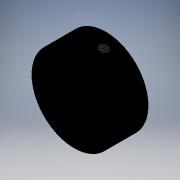
# Autodesk Inventor part: SCHUNK-Flansch IP 40 ERD
Saved by Autodesk Inventor 2017.3 (Build 213256000, 256)
## iProperties
Part Number: SCHUNK-Flansch IP 40 ERD
Material: Generic
Catalog Web Link: www.cadenas.de
Description: Flansch ERD-Miniature rotary unit
Vendor: SCHUNK
Document SubType Name: Modeling
Designer: partserver
Manufacturer: SCHUNK
Mass: 46.2323 g
Surface Area: 96.2708 cm^2
Volume: 46.2323 cm^3
Density: 1 g/cm^3
Appearance: PSOLRGB-0-0-0
Category: PARTsolutions
Company: SCHUNK
Title: SCHUNK-Flansch IP 40 ERD
Author: Cadenas PARTsolutions
Comments: Miniature rotary unit
PSOL_IDENT_0: {$CADENAS_DATA\23d-libs\schunk\greifsysteme\drehmodule\drehmodule_elektrisch\schwenkeinheiten\miniat
PSOL_IDENT_1: ur_schwenkeinheiten\erd_welle.prj},193 {VTYP=3D},{NB=SCHUNK-Flansch IP 40 ERD},{LINA=SCHUNK-Flansch
PSOL_IDENT_2: IP 40 ERD},{NN=Flansch ERD},{DATE=23.04.2020 15:23:31},{GEOMDATE=04.12.2019 08:06:04},{VERSION=},{LI
PSOL_IDENT_3: NEID=20},{WBVAR=},{WBNUMERIC=}  {NB=SCHUNK-Flansch IP 40 ERD},{LINA=SCHUNK-Flansch IP 40 ERD},{KT=DU
PSOL_IDENT_4: MMY},{TYP=Flansch IP 40},{KD1=55.000},{KD2=25.000},{KH1=20.500},{KH2=2.000},{BA1=28.300},{BA2=20.000
PSOL_IDENT_5: },{BA3=11.000},{BD1=5.000},{BD2=5.000},{BD3=10.000},{BD4=4.200},{BD5=2.500},{BT1=11.000},{BT2=5.000}
PSOL_IDENT_6: ,{BT3=0.700},{BT4=2.500},{BA4=20.500},{BA5=12.500},{BD6=10.000},{BD7=7.000},{BT6=0.500},{BT7=5.000},
PSOL_IDENT_7: {BW=15.000},{SBD=2.500},{SBW=4.000},{SBA1=8.500},{SBA2=22.700},{SBA3=13.000},{SBT1=10.400},{SBT2=22.
PSOL_IDENT_8: 900},{TYP1=40.000}
NB: SCHUNK-Flansch IP 40 ERD
NN: Flansch ERD
NT: Miniature rotary unit
NBSYN: SCHUNK-$TYP. ERD
LINA: SCHUNK-Flansch IP 40 ERD
CATALOG: SCHUNK
TYP: Flansch IP 40
KD1: 55
KD2: 25
KH1: 20.5
KH2: 2
BA1: 28.3
BA2: 20
BA3: 11
BD1: 5
BD2: 5
BD3: 10
BD4: 4.2
BD5: 2.5
BT1: 11
BT2: 5
BT3: 0.7
BT4: 2.5
BA4: 20.5
BA5: 12.5
BD6: 10
BD7: 7
BT6: 0.5
BT7: 5
BW: 15
SBD: 2.5
SBW: 4
SBA1: 8.5
SBA2: 22.7
SBA3: 13
SBT1: 10.4
SBT2: 22.9
TYP1: 40
SUPPLIER: SCHUNK
ARTICLENO: SCHUNK-Flansch IP 40 ERD
BOMINFO: SCHUNK-Flansch IP 40 ERD
CREATOR: CADENAS GmbH
Autodesk Inventor part; units mm, degrees
sketch "Sketch_1" plane through (0, 0, 0) normal (0, 0, 1) x (1, 0, 0)
  line L0 (0, 0) -> (0, 20)
  line L1 (0, 18.5) -> (12.5, 18.5)
  line L2 (12.5, 18.5) -> (12.5, 20.2)
  line L3 (12.5, 20.2) -> (12.8, 20.5)
  line L4 (12.8, 20.5) -> (27.5, 20.5)
  line L5 (27.5, 20.5) -> (27.5, 0)
  line L6 (27.5, 0) -> (0, 0)
  line L7 (0, 0) -> (0, 18.5)
  constraints: 16 end point
revolve "Revolution1" add sketch "Sketch_1" angle 360 about axis through (0, 0, 0) along (0, -1, 0)
sketch "Sketch_2" plane through (0, 0, 0) normal (1, 0, 0) x (0, 1, 0)
  line L0 (18.5, 5.5) -> (14.5489, 5.5)
  line L1 (14.5489, 5.5) -> (15.3, 6.75)
  line L2 (15.3, 6.75) -> (17.6, 6.75)
  line L3 (17.6, 6.75) -> (17.8, 6.95)
  line L4 (17.8, 6.95) -> (17.8, 7.4)
  line L5 (17.8, 7.4) -> (17.6, 7.6)
  line L6 (17.6, 7.6) -> (17.8, 7.6)
  line L7 (17.8, 7.6) -> (17.8, 10.5)
  line L8 (17.8, 10.5) -> (18.5, 10.5)
  line L9 (18.5, 10.5) -> (18.5, 5.5)
  line L10 (18.5, 5.5) -> (14.5489, 5.5)
  constraints: 22 end point
revolve "Revolution2" cut sketch "Sketch_2" angle 360 about axis through (0, 18.5, 5.5) along (0, 1, 0)
pattern_linear "Rectangular Pattern1" count 2 spacing 11 along (0, 0, -1) of "Revolution2"
sketch "Sketch_7" plane through (0, 17.8, 5.5) normal (0, 1, 0) x (0, 0, 1)
  line L0 (-1.25, -0.7217) -> (0, -1.4434)
  line L1 (0, -1.4434) -> (1.25, -0.7217)
  line L2 (1.25, -0.7217) -> (1.25, 0.7217)
  line L3 (1.25, 0.7217) -> (0, 1.4434)
  line L4 (0, 1.4434) -> (-1.25, 0.7217)
  line L5 (-1.25, 0.7217) -> (-1.25, -0.7217)
  constraints: 12 end point
extrude "Extrusion1" cut sketch "Sketch_7" against normal blind 2.5
pattern_linear "Rectangular Pattern2" count 2 spacing 11 along (0, 0, -1) of "Extrusion1"
sketch "Sketch4" plane through (0, 20.5, 0) normal (0, 1, 0) x (1, 0, 0)
  point P0 (-14.1421, 14.1421)
hole "Hole1" at (-14.1421, 20.5, -14.1421) direction (0, -1, 0) diameter 4.134 depth 11 tip angle 120 countersink diameter 5 countersink angle 90 thread size "M5x0.8" class "6H" standard "ISO Metric profile"
pattern_linear "Rectangular Pattern3" count 2 spacing 28.2843 along (1, 0, 0) count 2 spacing 28.2843 along (0, 0, 1) of "Hole1"
sketch "Sketch5" plane through (0, 20.5, 0) normal (0, 1, 0) x (1, 0, 0)
  point P0 (-20, 0)
hole "Hole2" at (-20, 20.5, 0) direction (0, -1, 0) diameter 5 depth 5 tip angle 118
sketch "Sketch_9" plane through (0, 12.5, 0) normal (0, 1, 0) x (1, 0, 0)
  line L0 (0, -18.397) -> (0, -27.5)
  line L1 (0, -27.5) -> (-5, -27.5)
  line L2 (-5, -27.5) -> (-5, -26.5)
  line L3 (-5, -26.5) -> (-2.9585, -26.5)
  line L4 (-2.9585, -26.5) -> (-2.9585, -20.1746)
  line L5 (-2.9585, -20.1746) -> (0, -18.397)
  line L6 (0, -18.397) -> (0, -27.5)
  constraints: 14 end point
revolve "Revolution3" cut sketch "Sketch_9" angle 360 about axis through (0, 12.5, 18.397) along (0, 0, -1)
thread "Thread1" size "M7x1" class "6H" standard "ISO Metric profile" length 6
sketch "Sketch_10" plane through (0, 12.5, 0) normal (0, 1, 0) x (1, 0, 0)
  line L0 (-4.7615, 17.7701) -> (-7.1175, 26.563)
  line L1 (-7.1175, 26.563) -> (-2.2879, 27.8571)
  line L2 (-2.2879, 27.8571) -> (-2.0291, 26.8911)
  line L3 (-2.0291, 26.8911) -> (-4.001, 26.3628)
  line L4 (-4.001, 26.3628) -> (-2.3639, 20.2529)
  line L5 (-2.3639, 20.2529) -> (-4.7615, 17.7701)
  line L6 (-4.7615, 17.7701) -> (-7.1175, 26.563)
  constraints: 14 end point
revolve "Revolution4" cut sketch "Sketch_10" angle 360 about axis through (-4.7615, 12.5, -17.7701) along (0.258819, 0, 0.9659258)
thread "Thread2" size "M7x1" class "6H" standard "ISO Metric profile" length 6
sketch "Sketch_11" plane through (0, 13, 0) normal (0, 1, 0) x (1, 0, 0)
  line L0 (27.433, 20.7817) -> (3.8395, 22.4315)
  line L1 (3.8395, 22.4315) -> (4.676, 23.6261)
  line L2 (4.676, 23.6261) -> (27.5202, 22.0287)
  line L3 (27.5202, 22.0287) -> (27.433, 20.7817)
  line L4 (27.433, 20.7817) -> (3.8395, 22.4315)
  constraints: 10 end point
revolve "Revolution5" cut sketch "Sketch_11" angle 360 about axis through (27.433, 13, -20.7817) along (0.9975641, 0, 0.0697565)
sketch "Sketch_12" plane through (0, 13, 0) normal (0, 1, 0) x (1, 0, 0)
  line L0 (27.433, 12.2817) -> (16.3091, 13.0596)
  line L1 (16.3091, 13.0596) -> (17.1455, 14.2541)
  line L2 (17.1455, 14.2541) -> (27.5202, 13.5287)
  line L3 (27.5202, 13.5287) -> (27.433, 12.2817)
  line L4 (27.433, 12.2817) -> (16.3091, 13.0596)
  constraints: 10 end point
revolve "Revolution6" cut sketch "Sketch_12" angle 360 about axis through (27.433, 13, -12.2817) along (0.9975641, 0, 0.0697565)
ref_plane "ring_stk_XY" through (0, 0, 0) normal (0, 1, 0) x (1, 0, 0)
ref_plane "ring_stk_YZ" through (0, 0, 0) normal (1, 0, 0) x (0, 0, -1)
ref_plane "ring_stk_ZX" through (0, 0, 0) normal (0, 0, -1) x (0, 1, 0)
ref_plane "stecker_XY" through (0, 13, 0) normal (0, 1, 0) x (1, 0, 0)
ref_plane "stecker_YZ" through (0, 13, 0) normal (1, 0, 0) x (0, 0, -1)
ref_plane "stecker_ZX" through (0, 13, 0) normal (0, 0, -1) x (0, 1, 0)
ref_plane "vss1_XY" through (0, 12.5, 26.5) normal (0, 0, 1) x (-1, 0, 0)
ref_plane "vss1_YZ" through (0, 12.5, 26.5) normal (-1, 0, 0) x (0, -1, 0)
ref_plane "vss1_ZX" through (0, 12.5, 26.5) normal (0, -1, 0) x (0, 0, 1)
ref_plane "vss2_XY" through (-6.8587, 12.5, -25.597) normal (-0.258819, 0, -0.9659258) x (0.9659258, 0, -0.258819)
ref_plane "vss2_YZ" through (-6.8587, 12.5, -25.597) normal (0.9659258, 0, -0.258819) x (0, -1, 0)
ref_plane "vss2_ZX" through (-6.8587, 12.5, -25.597) normal (0, -1, 0) x (-0.258819, 0, -0.9659258)
body "Solid1"
